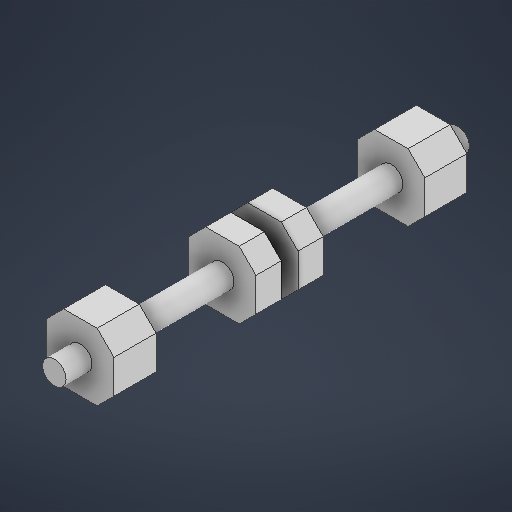
# Autodesk Inventor part: EjeFrontalGrúa
Saved by Autodesk Inventor 2026.2 (Build 302298010, 298A)
## iProperties
Created: 2026-04-23
Part Number: EjeFrontalGrúa
Material: Genérico
Document SubType Name: Modeling
Designer: Jose Carlos
Density: 1 g/cm^3
Appearance: Valor por defecto
Author: Jose Carlos
Autodesk Inventor part; units mm, degrees
ref_plane "Plano de trabajo1" through (0, 0, 0) normal (0, 0, 1) x (1, 0, 0)
sketch "Boceto1" plane through (0, 0, 0) normal (0, 0, 1) x (1, 0, 0)
  circle A0 centre (-38.2477, 31.5) radius 1.5 construction
  circle A1 centre (-38.2477, 31.5) radius 1.4
  point P0 (0, 0)
  dimension "d2" = 0.1
  constraints: 1 centre point, 1 coincident
  measures "d2" radial gap between concentric circles of A0 A1
ref_plane "Plano de trabajo2" through (-44.5, -51.5, -48) normal (0, 0, -1) x (0, 1, 0)
extrude "Extrusión1" add sketch "Boceto1" against normal up to surface (48 mm away)
ref_plane "Plano de trabajo3" through (0, 0, -45.1) normal (0, 0, 1) x (1, 0, 0)
sketch "Boceto2" plane through (0, 0, -45.1) normal (0, 0, 1) x (1, 0, 0)
  circle A0 centre (-38.2477, 31.5) radius 1.4 construction
  line L0 (-34.2477, 35.5) -> (-42.2477, 35.5)
  line L1 (-42.2477, 35.5) -> (-42.2477, 27.5)
  line L2 (-42.2477, 27.5) -> (-34.2477, 27.5)
  line L3 (-34.2477, 27.5) -> (-34.2477, 35.5)
  line L4 (-34.2477, 35.5) -> (-42.2477, 27.5) construction
  line L5 (-42.2477, 35.5) -> (-34.2477, 27.5) construction
  point P0 (0, 0)
  dimension "d3" = 8
  dimension "d4" = 8
  constraints: 12 end point, 2 midpoint, 2 parallel, 1 horizontal, 1 perpendicular
  measures "d3" distance of L1.end L2.end
  measures "d4" distance of L0.end L1.end
extrude "Extrusión2" add sketch "Boceto2" along normal blind 5
chamfer "Chaflán1" distance 2 angle 45 4 edges at (-42.2477, 35.5, -42.6) (-34.2477, 35.5, -42.6) (-34.2477, 27.5, -42.6) (-42.2477, 27.5, -42.6)
ref_plane "Plano de trabajo4" through (0, 0, -3.1) normal (0, 0, -1) x (-1, 0, 0)
sketch "Boceto3" plane through (0, 0, -3.1) normal (0, 0, -1) x (-1, 0, 0)
  circle A0 centre (38.2477, 31.5) radius 1.4 construction
  line L0 (34.2477, 27.5) -> (42.2477, 27.5)
  line L1 (42.2477, 27.5) -> (42.2477, 35.5)
  line L2 (42.2477, 35.5) -> (34.2477, 35.5)
  line L3 (34.2477, 35.5) -> (34.2477, 27.5)
  line L4 (34.2477, 27.5) -> (42.2477, 35.5) construction
  line L5 (42.2477, 27.5) -> (34.2477, 35.5) construction
  point P0 (0, 0)
  dimension "d10" = 8
  dimension "d11" = 8
  constraints: 12 end point, 2 midpoint, 2 parallel, 1 horizontal, 1 perpendicular
  measures "d10" distance of L0.end L1.end
  measures "d11" distance of L0.start L0.end
extrude "Extrusión3" add sketch "Boceto3" along normal blind 5
chamfer "Chaflán2" distance 2 angle 45 4 edges at (-42.2477, 35.5, -5.6) (-34.2477, 35.5, -5.6) (-34.2477, 27.5, -5.6) (-42.2477, 27.5, -5.6)
ref_plane "Plano de trabajo5" through (-38.2477, 31.5, -24) normal (0, 0, -1) x (-1, 0, 0)
sketch "Boceto4" plane through (-38.2477, 31.5, -24) normal (0, 0, -1) x (-1, 0, 0)
  circle A0 centre (0, 0) radius 1.5 construction
  line L0 (-4, -4) -> (4, -4)
  line L1 (4, -4) -> (4, 4)
  line L2 (4, 4) -> (-4, 4)
  line L3 (-4, 4) -> (-4, -4)
  line L4 (-4, -4) -> (4, 4) construction
  line L5 (4, -4) -> (-4, 4) construction
  point P0 (-38.2477, -31.5)
  dimension "d17" = 8
  dimension "d18" = 8
  constraints: 12 end point, 2 midpoint, 2 parallel, 1 horizontal, 1 perpendicular
  measures "d17" distance of L0.end L1.end
  measures "d18" distance of L1.end L2.end
extrude "Extrusión4" add sketch "Boceto4" along normal mid plane 8
chamfer "Chaflán3" distance 2 angle 45 4 edges at (-42.2477, 35.5, -24) (-42.2477, 27.5, -24) (-34.2477, 35.5, -24) (-34.2477, 27.5, -24)
sketch "Boceto5" plane through (-38.2477, 31.5, -24) normal (0, 0, -1) x (-1, 0, 0)
  circle A0 centre (0, 0) radius 1.4 construction
  line L0 (-4, 4) -> (4, 4)
  line L1 (4, 4) -> (4, -4)
  line L2 (4, -4) -> (-4, -4)
  line L3 (-4, -4) -> (-4, 4)
  line L4 (-4, 4) -> (4, -4) construction
  line L5 (4, 4) -> (-4, -4) construction
  circle A1 centre (0, 0) radius 1.4
  point P0 (-38.2477, -31.5)
  dimension "d24" = 8
  dimension "d25" = 8
  constraints: 12 end point, 2 midpoint, 2 parallel, 1 centre point, 1 coincident, 1 concentric, 1 horizontal, 1 perpendicular
  measures "d24" distance of L0.end L1.end
  measures "d25" distance of L1.end L2.end
extrude "Extrusión5" cut sketch "Boceto5" along normal mid plane 2
